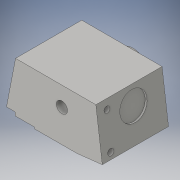
# Autodesk Inventor part: Gearbox
Saved by Autodesk Inventor 2016 (Build 200138000, 138)
## iProperties
Created: 2017-02-14
Part Number: Gearbox
Material: Generic
Document SubType Name: Modeling
Designer: m215104
Density: 1 g/cm^3
Appearance: Default
Author: m215104
Autodesk Inventor part; units mm, degrees
ref_plane "YZ Plane" through (0, 0, 0) normal (1, 0, 0) x (0, 1, 0)
ref_plane "XZ Plane" through (0, 0, 0) normal (0, 1, 0) x (-1, 0, 0)
ref_plane "XY Plane" through (0, 0, 0) normal (0, 0, 1) x (1, 0, 0)
sketch "Sketch1" plane through (0, 0, 0) normal (0, 0, 1) x (1, 0, 0)
  line L0 (0, 0) -> (220, 0)
  line L1 (110, 0) -> (110, 266.5) construction
  line L2 (110, 266.5) -> (317.5, 266.5)
  line L3 (110, 266.5) -> (-97.5, 266.5)
  line L4 (220, 0) -> (340, 0) construction
  line L5 (317.5, 266.5) -> (350.6537, 14.673)
  line L6 (317.5, 266.5) -> (571.5, 266.5) construction
  line L7 (350.6537, 14.673) -> (220, 0)
  line L8 (-97.5, 266.5) -> (-144.2482, 26.0013)
  line L9 (-97.5, 266.5) -> (147.5, 266.5) construction
  line L10 (-144.2482, 26.0013) -> (-101.2482, 26.0013)
  line L11 (-99.2482, 24.0013) -> (-99.2482, 8.0013)
  line L12 (-99.2482, 8.0013) -> (-2, 8.0013)
  line L13 (0, 6.0013) -> (0, 0)
  arc A0 (0, 6.0013) -> (-2, 8.0013) centre (-2, 6.0013) ccw
  arc A1 (-99.2482, 24.0013) -> (-101.2482, 26.0013) centre (-101.2482, 24.0013) ccw
  point P0 (-99.2482, 26.0013)
  dimension "d0" = 220
  dimension "d1" = 266.5
  dimension "d7" = 254
  dimension "d8" = 82.5
  dimension "d9" = 245
  dimension "d10" = 101
  dimension "d11" = 45
  dimension "d12" = 18
  dimension "d14" = 415
  dimension "d15" = 2
  dimension "d16" = 2
  constraints: 28 end point, 6 horizontal, 4 point on circle, 4 tangent, 2 centre point, 2 equal length, 2 perpendicular, 2 point on line, 1 midpoint, 1 parallel, 1 symmetric about line, 1 vertical
  measures "d0" distance of L0.start L0.end
  measures "d1" distance of L1.start L1.end
  measures "d7" distance of L2.end L5.end
  measures "d8" angle of L5 L6
  measures "d9" distance of L3.end L8.end
  measures "d10" angle of L8 L9
  measures "d11" distance of L8.end point (-99.248, 26.001)
  measures "d12" distance of point (-99.248, 26.001) L11.end
  measures "d14" distance of L2.end L3.end
  measures "d15" radius of A0
  measures "d16" radius of A1
extrude "Extrusion1" add sketch "Sketch1" along normal blind 342
sketch "Sketch3" plane through (317.5, 266.5, 342) normal (0.9914449, 0.1305262, 0) x (0, 0, -1)
  circle A0 centre (182, -91.5) radius 70
  line L0 (342, -254) -> (342, 0) projected
  line L1 (342, 0) -> (0, 0) projected
  line L2 (252, -91.5) -> (342, -91.5) construction
  line L3 (182, -21.5) -> (182, 0) construction
  point P0 (342, -222.778)
  dimension "d22" = 140
  dimension "d26" = 160
  dimension "d27" = 70
  dimension "d28" = 91.5
  dimension "d29" = 70
  constraints: 4 end point, 2 perpendicular, 2 point on circle, 2 point on line, 1 centre point
  measures "d22" diameter of A0
  measures "d26" distance from line of L2.end L3
  measures "d27" distance from line of L2.start L3
  measures "d28" distance from line of L3.end L2
  measures "d29" distance from line of L3.start L2
extrude "Extrusion2" cut sketch "Sketch3" against normal blind 10
sketch "Sketch4" plane through (317.5, 266.5, 342) normal (0.9914449, 0.1305262, 0) x (0, 0, -1)
  line L0 (342, 0) -> (0, 0) projected
  line L1 (0, -254) -> (0, 0) projected
  circle A0 centre (51, -45) radius 15
  line L2 (51, 0) -> (51, -45) construction
  line L3 (51, -45) -> (0, -45) construction
  circle A1 centre (47.75, -223.25) radius 15.75
  line L4 (342, -254) -> (0, -254) projected
  line L5 (47.75, -223.25) -> (0, -223.25) construction
  line L6 (47.75, -223.25) -> (47.75, -254) construction
  point P0 (342, -222.778)
  dimension "d34" = 30
  dimension "d37" = 45
  dimension "d38" = 51
  dimension "d39" = 31.5
  dimension "d42" = 30.75
  dimension "d43" = 47.75
  constraints: 8 end point, 4 point on line, 3 perpendicular, 2 centre point, 1 vertical
  measures "d34" diameter of A0
  measures "d37" distance of L2.start L2.end
  measures "d38" distance of L2.end L3.end
  measures "d39" diameter of A1
  measures "d42" distance of L5.start L6.end
  measures "d43" distance of L5.start L5.end
extrude "Extrusion3" cut sketch "Sketch4" against normal blind 60
sketch "Sketch5" plane through (0, 0, 0) normal (0, 0, -1) x (-1, 0, 0)
  line L0 (-350.6537, 14.673) -> (-317.5, 266.5) projected
  line L1 (-317.5, 266.5) -> (97.5, 266.5) projected
  circle A0 centre (-142.0425, 167.4324) radius 80.5
  line L2 (-142.0425, 247.9324) -> (-142.0425, 266.9324) construction
  line L3 (-142.0425, 167.4324) -> (-330.5425, 167.4324) construction
  point P0 (0, 0)
  dimension "d49" = 161
  dimension "d50" = 19
  dimension "d52" = 188.5
  constraints: 4 end point, 1 horizontal, 1 point on line, 1 vertical, 1 vertical alignment, 2 other
  measures "d50" distance of L2.start L2.end
  measures "d52" distance of L3.start L3.end
extrude "Extrusion4" add sketch "Sketch5" along normal blind 26
sketch "Sketch6" plane through (142.0425, 167.4324, -26) normal (0, 0, -1) x (-1, 0, 0)
  circle A0 centre (0, 0) radius 29
  point P0 (142.0425, -167.4324)
  dimension "d55" = 58
  constraints: 1 centre point
  measures "d55" diameter of A0
extrude "Extrusion5" cut sketch "Sketch6" against normal through all
sketch "Sketch7" plane through (0, 0, 0) normal (0, 0, -1) x (-1, 0, 0)
  line L0 (-39.1667, 56.5) -> (-35.7652, 56.5)
  line L1 (-45.3265, 16.5) -> (-29.6054, 16.5)
  line L2 (-48.9954, 48.3429) -> (-53.1895, 25.9743)
  line L3 (-25.9365, 48.3429) -> (-21.7424, 25.9743)
  arc A0 (-39.1667, 56.5) -> (-48.9954, 48.3429) centre (-39.1667, 46.5) ccw
  arc A1 (-25.9365, 48.3429) -> (-35.7652, 56.5) centre (-35.7652, 46.5) ccw
  arc A2 (-53.1895, 25.9743) -> (-45.3265, 16.5) centre (-45.3265, 24.5) ccw
  arc A3 (-29.6054, 16.5) -> (-21.7424, 25.9743) centre (-29.6054, 24.5) ccw
  line L4 (0, 0) -> (-220, 0) projected
  line L5 (-110, 0) -> (-110, 69.6289)
  line L6 (-180.8333, 56.5) -> (-184.2348, 56.5)
  line L7 (-174.6735, 16.5) -> (-190.3946, 16.5)
  line L8 (-171.0046, 48.3429) -> (-166.8105, 25.9743)
  line L9 (-194.0635, 48.3429) -> (-198.2576, 25.9743)
  arc A4 (-171.0046, 48.3429) -> (-180.8333, 56.5) centre (-180.8333, 46.5) ccw
  arc A5 (-184.2348, 56.5) -> (-194.0635, 48.3429) centre (-184.2348, 46.5) ccw
  arc A6 (-174.6735, 16.5) -> (-166.8105, 25.9743) centre (-174.6735, 24.5) ccw
  arc A7 (-198.2576, 25.9743) -> (-190.3946, 16.5) centre (-190.3946, 24.5) ccw
  point P0 (-47.466, 56.5)
  point P1 (-27.466, 56.5)
  point P2 (-54.966, 16.5)
  point P3 (-19.966, 16.5)
  point P4 (-172.534, 56.5)
  point P5 (-192.534, 56.5)
  point P6 (-165.034, 16.5)
  point P7 (-200.034, 16.5)
  dimension "d69" = 20
  dimension "d70" = 35
  dimension "d72" = 10
  dimension "d73" = 8
  constraints: 18 end point, 16 point on circle, 16 point on line, 16 symmetric about line, 8 centre point, 8 tangent, 2 equal radius, 2 horizontal, 1 midpoint, 1 vertical, 4 other
  measures "d69" distance of point (-47.466, 56.5) point (-27.466, 56.5)
  measures "d70" distance of point (-54.966, 16.5) point (-19.966, 16.5)
  measures "d72" radius of A0
  measures "d73" radius of A2
extrude "Extrusion6" cut sketch "Sketch7" against normal blind 6
fillet "Fillet1" radius 2 8 edges at (182.534, 56.5, 6) (174.447, 54.1951, 6) (168.9075, 37.1586, 6) (168.5174, 19.3909, 6) (182.534, 16.5, 6) (196.5507, 19.3909, 6) (196.1606, 37.1586, 6) (190.6211, 54.1951, 6)
fillet "Fillet2" radius 2 8 edges at (51.0925, 37.1586, 6) (45.553, 54.1951, 6) (37.466, 56.5, 6) (29.3789, 54.1951, 6) (23.8394, 37.1586, 6) (23.4493, 19.3909, 6) (37.466, 16.5, 6) (51.4826, 19.3909, 6)
body "Solid1"
